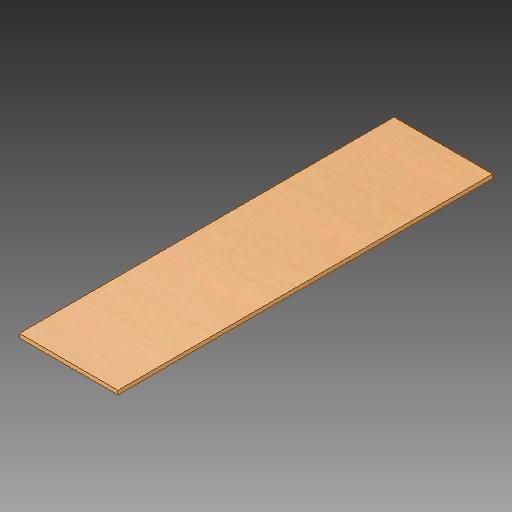
# Autodesk Inventor part: shelf
Saved by Autodesk Inventor 2019 (Build 230136000, 136)
## iProperties
Created: 2019-05-05
Part Number: shelf
Material: Madeira
Document SubType Name: Modeling
Designer: Daniel Regner
Density: 0.570257 g/cm^3
Appearance: Pinho amarelo - Sólido natural sem brilho
Author: Daniel Regner
Autodesk Inventor part; units mm, degrees
ref_plane "YZ Plane" through (0, 0, 0) normal (1, 0, 0) x (0, 1, 0)
ref_plane "XZ Plane" through (0, 0, 0) normal (0, 1, 0) x (-1, 0, 0)
ref_plane "XY Plane" through (0, 0, 0) normal (0, 0, 1) x (1, 0, 0)
sketch "Esboço1" plane through (0, 0, 0) normal (0, 1, 0) x (-1, 0, 0)
  line L0 (-125, -475) -> (125, -475)
  line L1 (125, -475) -> (125, 475)
  line L2 (125, 475) -> (-125, 475)
  line L3 (-125, 475) -> (-125, -475)
  line L4 (-125, -475) -> (125, 475) construction
  line L5 (125, -475) -> (-125, 475) construction
  point P0 (0, 0)
  dimension "d0" = 250
  dimension "d1" = 950
  constraints: 12 end point, 2 midpoint, 2 parallel, 1 horizontal, 1 perpendicular
  measures "d0" distance of L2.end L1.end
  measures "d1" distance of L1.end L0.end
extrude "Extrusão1" add sketch "Esboço1" along normal blind 10
equation "\"d1\" = LENGHT - 2 * RIP_L"
equation "\"RIP_L\" = 25"
equation "\"LENGHT\" = 1000"
